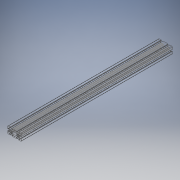
# Autodesk Inventor part: 1530-S
Saved by Autodesk Inventor 2019 (Build 230136000, 136)
## iProperties
Company: 80/20 Inc.
Created: 2013-09-06
Part Number: 1530-S
Material: Generic
Document SubType Name: Modeling
Density: 1 g/cm^3
Catalog Web Link: 8020.net
Vendor: 80/20 Inc.
Engineer: Ross Bowman
Appearance: Black
Author: Ross Bowman
Keywords: T-Slot, Extrusion, 80/20, 8020, Quick Frame, HT
Autodesk Inventor part; units mm, degrees
ref_plane "YZ Plane" through (0, 0, 0) normal (1, 0, 0) x (0, 1, 0)
ref_plane "XZ Plane" through (0, 0, 0) normal (0, 1, 0) x (-1, 0, 0)
ref_plane "XY Plane" through (0, 0, 0) normal (0, 0, 1) x (1, 0, 0)
sketch "Sketch1" plane through (0, 0, 0) normal (0, 0, 1) x (1, 0, 0)
  arc A0 (-21.6898, 4.2456) -> (-23.2956, 2.6398) centre (-22.5851, 3.5351) ccw
  line L0 (-20.4064, 2.9729) -> (-21.6898, 4.2456)
  arc A1 (-17.6936, 2.9729) -> (-20.4064, 2.9729) centre (-19.05, 0) ccw
  line L1 (-16.3231, 4.3433) -> (-17.6936, 2.9729)
  arc A2 (-14.7067, 2.7269) -> (-16.3231, 4.3433) centre (-15.5149, 3.5351) ccw
  line L2 (-16.0771, 1.3564) -> (-14.7067, 2.7269)
  arc A3 (-16.0771, -1.3564) -> (-16.0771, 1.3564) centre (-19.05, 0) ccw
  line L3 (-14.7067, -2.7269) -> (-16.0771, -1.3564)
  arc A4 (-16.3231, -4.3433) -> (-14.7067, -2.7269) centre (-15.5149, -3.5351) ccw
  line L4 (-17.6936, -2.9729) -> (-16.3231, -4.3433)
  arc A5 (-20.4064, -2.9729) -> (-17.6936, -2.9729) centre (-19.05, 0) ccw
  line L5 (-21.7769, -4.3433) -> (-20.4064, -2.9729)
  arc A6 (-23.3933, -2.7269) -> (-21.7769, -4.3433) centre (-22.5851, -3.5351) ccw
  line L6 (-22.0229, -1.3564) -> (-23.3933, -2.7269)
  arc A7 (-22.0229, 1.3564) -> (-22.0229, -1.3564) centre (-19.05, 0) ccw
  line L7 (-23.2956, 2.6398) -> (-22.0229, 1.3564)
  arc A8 (2.0655, 14.1109) -> (-2.0655, 14.1109) centre (0, 12.0454) ccw
  line L8 (10.7892, 5.3872) -> (2.0655, 14.1109)
  arc A9 (12.1803, 2.0285) -> (10.7892, 5.3872) centre (7.4305, 2.0285) ccw
  line L9 (12.1803, -2.0285) -> (12.1803, 2.0285)
  arc A10 (10.7892, -5.3872) -> (12.1803, -2.0285) centre (7.4305, -2.0285) ccw
  line L10 (2.0655, -14.1109) -> (10.7892, -5.3872)
  arc A11 (-2.0655, -14.1109) -> (2.0655, -14.1109) centre (0, -12.0454) ccw
  line L11 (-10.7892, -5.3872) -> (-2.0655, -14.1109)
  arc A12 (-12.1803, -2.0285) -> (-10.7892, -5.3872) centre (-7.4305, -2.0285) ccw
  line L12 (-12.1803, 2.0285) -> (-12.1803, -2.0285)
  arc A13 (-10.7892, 5.3872) -> (-12.1803, 2.0285) centre (-7.4305, 2.0285) ccw
  line L13 (-2.0655, 14.1109) -> (-10.7892, 5.3872)
  arc A14 (16.4102, 4.2456) -> (14.8044, 2.6398) centre (15.5149, 3.5351) ccw
  line L14 (17.6936, 2.9729) -> (16.4102, 4.2456)
  arc A15 (20.4064, 2.9729) -> (17.6936, 2.9729) centre (19.05, 0) ccw
  line L15 (21.7769, 4.3433) -> (20.4064, 2.9729)
  arc A16 (23.3933, 2.7269) -> (21.7769, 4.3433) centre (22.5851, 3.5351) ccw
  line L16 (22.0229, 1.3564) -> (23.3933, 2.7269)
  arc A17 (22.0229, -1.3564) -> (22.0229, 1.3564) centre (19.05, 0) ccw
  line L17 (23.3933, -2.7269) -> (22.0229, -1.3564)
  arc A18 (21.7769, -4.3433) -> (23.3933, -2.7269) centre (22.5851, -3.5351) ccw
  line L18 (20.4064, -2.9729) -> (21.7769, -4.3433)
  arc A19 (17.6936, -2.9729) -> (20.4064, -2.9729) centre (19.05, 0) ccw
  line L19 (16.3231, -4.3433) -> (17.6936, -2.9729)
  arc A20 (14.7067, -2.7269) -> (16.3231, -4.3433) centre (15.5149, -3.5351) ccw
  line L20 (16.0771, -1.3564) -> (14.7067, -2.7269)
  arc A21 (16.0771, 1.3564) -> (16.0771, -1.3564) centre (19.05, 0) ccw
  line L21 (14.8044, 2.6398) -> (16.0771, 1.3564)
  arc A22 (-24.6888, 14.986) -> (-23.114, 16.5608) centre (-24.6888, 16.5608) ccw
  line L22 (-23.114, 16.5608) -> (-23.114, 17.4752)
  arc A23 (-23.114, 17.4752) -> (-24.6888, 19.05) centre (-24.6888, 17.4752) ccw
  line L23 (-24.6888, 19.05) -> (-34.925, 19.05)
  arc A24 (-34.925, 19.05) -> (-38.1, 15.875) centre (-34.925, 15.875) ccw
  line L24 (-38.1, 15.875) -> (-38.1, 5.6388)
  arc A25 (-38.1, 5.6388) -> (-36.5252, 4.064) centre (-36.5252, 5.6388) ccw
  line L25 (-36.5252, 4.064) -> (-35.6108, 4.064)
  arc A26 (-35.6108, 4.064) -> (-34.036, 5.6388) centre (-35.6108, 5.6388) ccw
  line L26 (-34.036, 5.6388) -> (-34.036, 9.398)
  arc A27 (-33.147, 10.287) -> (-34.036, 9.398) centre (-33.147, 9.398) ccw
  line L27 (-33.147, 10.287) -> (-32.5789, 10.287)
  arc A28 (-31.9503, 10.0266) -> (-32.5789, 10.287) centre (-32.5789, 9.398) ccw
  line L28 (-31.9503, 10.0266) -> (-27.3108, 5.3872)
  arc A29 (-25.9197, 2.0285) -> (-27.3108, 5.3872) centre (-30.6695, 2.0285) ccw
  line L29 (-25.9197, 2.0285) -> (-25.9197, -2.0285)
  arc A30 (-27.3108, -5.3872) -> (-25.9197, -2.0285) centre (-30.6695, -2.0285) ccw
  line L30 (-27.3108, -5.3872) -> (-31.9503, -10.0266)
  arc A31 (-32.5789, -10.287) -> (-31.9503, -10.0266) centre (-32.5789, -9.398) ccw
  line L31 (-32.5789, -10.287) -> (-33.147, -10.287)
  arc A32 (-34.036, -9.398) -> (-33.147, -10.287) centre (-33.147, -9.398) ccw
  line L32 (-34.036, -9.398) -> (-34.036, -5.6388)
  arc A33 (-34.036, -5.6388) -> (-35.6108, -4.064) centre (-35.6108, -5.6388) ccw
  line L33 (-35.6108, -4.064) -> (-36.5252, -4.064)
  arc A34 (-36.5252, -4.064) -> (-38.1, -5.6388) centre (-36.5252, -5.6388) ccw
  line L34 (-38.1, -5.6388) -> (-38.1, -15.875)
  arc A35 (-38.1, -15.875) -> (-34.925, -19.05) centre (-34.925, -15.875) ccw
  line L35 (-34.925, -19.05) -> (-24.6888, -19.05)
  arc A36 (-24.6888, -19.05) -> (-23.114, -17.4752) centre (-24.6888, -17.4752) ccw
  line L36 (-23.114, -17.4752) -> (-23.114, -16.5608)
  arc A37 (-23.114, -16.5608) -> (-24.6888, -14.986) centre (-24.6888, -16.5608) ccw
  line L37 (-24.6888, -14.986) -> (-28.448, -14.986)
  arc A38 (-29.337, -14.097) -> (-28.448, -14.986) centre (-28.448, -14.097) ccw
  line L38 (-29.337, -14.097) -> (-29.337, -13.5289)
  arc A39 (-29.0766, -12.9003) -> (-29.337, -13.5289) centre (-28.448, -13.5289) ccw
  line L39 (-29.0766, -12.9003) -> (-24.4372, -8.2608)
  arc A40 (-21.0785, -6.8697) -> (-24.4372, -8.2608) centre (-21.0785, -11.6195) ccw
  line L40 (-21.0785, -6.8697) -> (-17.0215, -6.8697)
  arc A41 (-13.6628, -8.2608) -> (-17.0215, -6.8697) centre (-17.0215, -11.6195) ccw
  line L41 (-13.6628, -8.2608) -> (-9.0234, -12.9003)
  arc A42 (-8.763, -13.5289) -> (-9.0234, -12.9003) centre (-9.652, -13.5289) ccw
  line L42 (-8.763, -13.5289) -> (-8.763, -14.097)
  arc A43 (-9.652, -14.986) -> (-8.763, -14.097) centre (-9.652, -14.097) ccw
  line L43 (-9.652, -14.986) -> (-13.4112, -14.986)
  arc A44 (-13.4112, -14.986) -> (-14.986, -16.5608) centre (-13.4112, -16.5608) ccw
  line L44 (-14.986, -16.5608) -> (-14.986, -17.4752)
  arc A45 (-14.986, -17.4752) -> (-13.4112, -19.05) centre (-13.4112, -17.4752) ccw
  line L45 (-13.4112, -19.05) -> (13.4112, -19.05)
  arc A46 (13.4112, -19.05) -> (14.986, -17.4752) centre (13.4112, -17.4752) ccw
  line L46 (14.986, -17.4752) -> (14.986, -16.5608)
  arc A47 (14.986, -16.5608) -> (13.4112, -14.986) centre (13.4112, -16.5608) ccw
  line L47 (13.4112, -14.986) -> (9.652, -14.986)
  arc A48 (8.763, -14.097) -> (9.652, -14.986) centre (9.652, -14.097) ccw
  line L48 (8.763, -14.097) -> (8.763, -13.5289)
  arc A49 (9.0234, -12.9003) -> (8.763, -13.5289) centre (9.652, -13.5289) ccw
  line L49 (9.0234, -12.9003) -> (13.6628, -8.2608)
  arc A50 (17.0215, -6.8697) -> (13.6628, -8.2608) centre (17.0215, -11.6195) ccw
  line L50 (17.0215, -6.8697) -> (21.0785, -6.8697)
  arc A51 (24.4372, -8.2608) -> (21.0785, -6.8697) centre (21.0785, -11.6195) ccw
  line L51 (24.4372, -8.2608) -> (29.0766, -12.9003)
  arc A52 (29.337, -13.5289) -> (29.0766, -12.9003) centre (28.448, -13.5289) ccw
  line L52 (29.337, -13.5289) -> (29.337, -14.097)
  arc A53 (28.448, -14.986) -> (29.337, -14.097) centre (28.448, -14.097) ccw
  line L53 (28.448, -14.986) -> (24.6888, -14.986)
  arc A54 (24.6888, -14.986) -> (23.114, -16.5608) centre (24.6888, -16.5608) ccw
  line L54 (23.114, -16.5608) -> (23.114, -17.4752)
  arc A55 (23.114, -17.4752) -> (24.6888, -19.05) centre (24.6888, -17.4752) ccw
  line L55 (24.6888, -19.05) -> (34.925, -19.05)
  arc A56 (34.925, -19.05) -> (38.1, -15.875) centre (34.925, -15.875) ccw
  line L56 (38.1, -15.875) -> (38.1, -5.6388)
  arc A57 (38.1, -5.6388) -> (36.5252, -4.064) centre (36.5252, -5.6388) ccw
  line L57 (36.5252, -4.064) -> (35.6108, -4.064)
  arc A58 (35.6108, -4.064) -> (34.036, -5.6388) centre (35.6108, -5.6388) ccw
  line L58 (34.036, -5.6388) -> (34.036, -9.398)
  arc A59 (33.147, -10.287) -> (34.036, -9.398) centre (33.147, -9.398) ccw
  line L59 (33.147, -10.287) -> (32.5789, -10.287)
  arc A60 (31.9503, -10.0266) -> (32.5789, -10.287) centre (32.5789, -9.398) ccw
  line L60 (31.9503, -10.0266) -> (27.3108, -5.3872)
  arc A61 (25.9197, -2.0285) -> (27.3108, -5.3872) centre (30.6695, -2.0285) ccw
  line L61 (25.9197, -2.0285) -> (25.9197, 2.0285)
  arc A62 (27.3108, 5.3872) -> (25.9197, 2.0285) centre (30.6695, 2.0285) ccw
  line L62 (27.3108, 5.3872) -> (31.9503, 10.0266)
  arc A63 (32.5789, 10.287) -> (31.9503, 10.0266) centre (32.5789, 9.398) ccw
  line L63 (32.5789, 10.287) -> (33.147, 10.287)
  arc A64 (34.036, 9.398) -> (33.147, 10.287) centre (33.147, 9.398) ccw
  line L64 (34.036, 9.398) -> (34.036, 5.6388)
  arc A65 (34.036, 5.6388) -> (35.6108, 4.064) centre (35.6108, 5.6388) ccw
  line L65 (35.6108, 4.064) -> (36.5252, 4.064)
  arc A66 (36.5252, 4.064) -> (38.1, 5.6388) centre (36.5252, 5.6388) ccw
  line L66 (38.1, 5.6388) -> (38.1, 15.875)
  arc A67 (38.1, 15.875) -> (34.925, 19.05) centre (34.925, 15.875) ccw
  line L67 (34.925, 19.05) -> (24.6888, 19.05)
  arc A68 (24.6888, 19.05) -> (23.114, 17.4752) centre (24.6888, 17.4752) ccw
  line L68 (23.114, 17.4752) -> (23.114, 16.5608)
  arc A69 (23.114, 16.5608) -> (24.6888, 14.986) centre (24.6888, 16.5608) ccw
  line L69 (24.6888, 14.986) -> (28.448, 14.986)
  arc A70 (29.337, 14.097) -> (28.448, 14.986) centre (28.448, 14.097) ccw
  line L70 (29.337, 14.097) -> (29.337, 13.5289)
  arc A71 (29.0766, 12.9003) -> (29.337, 13.5289) centre (28.448, 13.5289) ccw
  line L71 (29.0766, 12.9003) -> (24.4372, 8.2608)
  arc A72 (21.0785, 6.8697) -> (24.4372, 8.2608) centre (21.0785, 11.6195) ccw
  line L72 (21.0785, 6.8697) -> (17.0215, 6.8697)
  arc A73 (13.6628, 8.2608) -> (17.0215, 6.8697) centre (17.0215, 11.6195) ccw
  line L73 (13.6628, 8.2608) -> (9.0234, 12.9003)
  arc A74 (8.763, 13.5289) -> (9.0234, 12.9003) centre (9.652, 13.5289) ccw
  line L74 (8.763, 13.5289) -> (8.763, 14.097)
  arc A75 (9.652, 14.986) -> (8.763, 14.097) centre (9.652, 14.097) ccw
  line L75 (9.652, 14.986) -> (13.4112, 14.986)
  arc A76 (13.4112, 14.986) -> (14.986, 16.5608) centre (13.4112, 16.5608) ccw
  line L76 (14.986, 16.5608) -> (14.986, 17.4752)
  arc A77 (14.986, 17.4752) -> (13.4112, 19.05) centre (13.4112, 17.4752) ccw
  line L77 (13.4112, 19.05) -> (-13.4112, 19.05)
  arc A78 (-13.4112, 19.05) -> (-14.986, 17.4752) centre (-13.4112, 17.4752) ccw
  line L78 (-14.986, 17.4752) -> (-14.986, 16.5608)
  arc A79 (-14.986, 16.5608) -> (-13.4112, 14.986) centre (-13.4112, 16.5608) ccw
  line L79 (-13.4112, 14.986) -> (-9.652, 14.986)
  arc A80 (-8.763, 14.097) -> (-9.652, 14.986) centre (-9.652, 14.097) ccw
  line L80 (-8.763, 14.097) -> (-8.763, 13.5289)
  arc A81 (-9.0234, 12.9003) -> (-8.763, 13.5289) centre (-9.652, 13.5289) ccw
  line L81 (-9.0234, 12.9003) -> (-13.6628, 8.2608)
  arc A82 (-17.0215, 6.8697) -> (-13.6628, 8.2608) centre (-17.0215, 11.6195) ccw
  line L82 (-17.0215, 6.8697) -> (-21.0785, 6.8697)
  arc A83 (-24.4372, 8.2608) -> (-21.0785, 6.8697) centre (-21.0785, 11.6195) ccw
  line L83 (-24.4372, 8.2608) -> (-29.0766, 12.9003)
  arc A84 (-29.337, 13.5289) -> (-29.0766, 12.9003) centre (-28.448, 13.5289) ccw
  line L84 (-29.337, 13.5289) -> (-29.337, 14.097)
  arc A85 (-28.448, 14.986) -> (-29.337, 14.097) centre (-28.448, 14.097) ccw
  line L85 (-28.448, 14.986) -> (-24.6888, 14.986)
  point P0 (0, 0)
  constraints: 172 end point, 172 point on circle, 86 centre point
extrude "Extrusion1" add sketch "Sketch1" against normal blind 838.2
body "Solid1"
